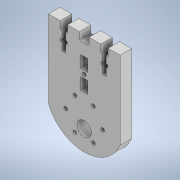
# Autodesk Inventor part: Крепление_мотора1_платформа
Saved by Autodesk Inventor 2020 (Build 240168000, 168)
## iProperties
Created: 2022-02-01
Part Number: Крепление_мотора1_платформа
Material: Типовые
Document SubType Name: Modeling
Designer: Администратор
Density: 1 g/cm^3
Appearance: По умолчанию
Autodesk Inventor part; units mm, degrees
ref_plane "YZ Plane" through (0, 0, 0) normal (1, 0, 0) x (0, 1, 0)
ref_plane "XZ Plane" through (0, 0, 0) normal (0, 1, 0) x (-1, 0, 0)
ref_plane "XY Plane" through (0, 0, 0) normal (0, 0, 1) x (1, 0, 0)
sketch "0" plane through (0, 0, 0) normal (0, 0, 1) x (1, 0, 0)
  line L0 (4.1594, 49.6005) -> (4.1594, 55.8505)
  line L1 (4.1594, 55.8505) -> (14.5761, 55.8505)
  line L2 (14.5761, 55.8505) -> (14.5761, 49.6005)
  line L3 (20.8261, 49.6005) -> (19.2636, 49.6005)
  line L4 (19.2636, 49.6005) -> (19.2636, 43.09)
  line L5 (19.2636, 33.9755) -> (16.1386, 33.9755)
  line L6 (16.1386, 33.9755) -> (16.1386, 40.4859)
  line L7 (14.8365, 43.09) -> (16.1386, 43.09)
  line L8 (20.5657, 43.09) -> (20.5657, 40.4859)
  line L9 (20.5657, 40.4859) -> (19.2636, 40.4859)
  line L10 (14.8365, 40.4859) -> (14.8365, 43.09)
  line L11 (16.1386, 43.09) -> (16.1386, 49.6005)
  line L12 (16.1386, 40.4859) -> (14.8365, 40.4859)
  line L13 (19.2636, 43.09) -> (20.5657, 43.09)
  line L14 (16.1386, 49.6005) -> (14.5761, 49.6005)
  line L15 (20.8261, 55.8505) -> (31.2428, 55.8505)
  line L16 (20.8261, 49.6005) -> (20.8261, 55.8505)
  line L17 (31.2428, 55.8505) -> (31.2428, 49.6005)
  line L18 (19.2636, 40.4859) -> (19.2636, 33.9755)
  line L19 (-31.2572, 49.6005) -> (-31.2572, 55.8505)
  line L20 (-31.2572, 55.8505) -> (-20.8406, 55.8505)
  line L21 (-14.5906, 55.8505) -> (-4.1739, 55.8505)
  line L22 (-4.1739, 55.8505) -> (-4.1739, 49.6005)
  line L23 (-3.1322, 49.6005) -> (-4.1739, 49.6005)
  line L24 (3.1178, 49.6005) -> (4.1594, 49.6005)
  line L25 (-20.8406, 55.8505) -> (-20.8406, 49.6005)
  line L26 (-14.5906, 49.6005) -> (-16.1531, 49.6005)
  line L27 (-16.1531, 49.6005) -> (-16.1531, 43.09)
  line L28 (-16.1531, 33.9755) -> (-19.2781, 33.9755)
  line L29 (-19.2781, 33.9755) -> (-19.2781, 40.4859)
  line L30 (-20.5802, 43.09) -> (-19.2781, 43.09)
  line L31 (-14.851, 43.09) -> (-14.851, 40.4859)
  line L32 (-14.851, 40.4859) -> (-16.1531, 40.4859)
  line L33 (-20.5802, 40.4859) -> (-20.5802, 43.09)
  line L34 (-19.2781, 43.09) -> (-19.2781, 49.6005)
  line L35 (-19.2781, 40.4859) -> (-20.5802, 40.4859)
  line L36 (-16.1531, 43.09) -> (-14.851, 43.09)
  line L37 (-19.2781, 49.6005) -> (-20.8406, 49.6005)
  line L38 (-14.5906, 49.6005) -> (-14.5906, 55.8505)
  line L39 (-16.1531, 40.4859) -> (-16.1531, 33.9755)
  arc A0 (-31.2572, -12.3787) -> (31.2428, -12.3787) centre (-0.0072, 0.6421) ccw
  circle A1 centre (8.0657, 5.7707) radius 1.5625
  circle A2 centre (-8.0802, 5.7707) radius 1.5625
  circle A3 centre (-16.1531, -8.212) radius 1.5625
  circle A4 centre (-8.0802, -22.1948) radius 1.5625
  circle A5 centre (8.0657, -22.1948) radius 1.5625
  circle A6 centre (16.1386, -8.212) radius 1.5625
  circle A7 centre (-0.0072, -15.5037) radius 6.25
  line L40 (31.2428, 49.6005) -> (31.2428, -12.3787)
  line L41 (-31.2572, -12.3787) -> (-31.2572, 49.6005)
  line L42 (-3.1322, 12.1005) -> (-3.1322, 22.5171)
  line L43 (-3.1322, 22.5171) -> (3.1178, 22.5171)
  line L44 (3.1178, 22.5171) -> (3.1178, 12.1005)
  line L45 (3.1178, 12.1005) -> (-3.1322, 12.1005)
  line L46 (-3.1322, 28.7671) -> (-3.1322, 39.1838)
  line L47 (3.1178, 39.1838) -> (3.1178, 28.7671)
  line L48 (3.1178, 28.7671) -> (-3.1322, 28.7671)
  circle A8 centre (-0.0072, 25.6421) radius 1.6667
  line L49 (-3.1322, 39.1838) -> (3.1178, 39.1838)
  line L50 (-3.1322, 49.6005) -> (3.1178, 49.6005)
  dimension "d0" = 12.5
  constraints: 102 end point, 9 centre point, 2 point on circle
  measures "d0" diameter of A7
sketch "Эскиз3" plane through (0, 0, 0) normal (0, 0, 1) x (1, 0, 0)
  circle A0 centre (-0.0072, -15.5037) radius 6.25
  circle A1 centre (-16.1531, -8.212) radius 1.5625
  circle A2 centre (-8.0802, 5.7707) radius 1.5625
  circle A3 centre (8.0657, 5.7707) radius 1.5625
  circle A4 centre (16.1386, -8.212) radius 1.5625
  circle A5 centre (8.0657, -22.1948) radius 1.5625
  circle A6 centre (-8.0802, -22.1948) radius 1.5625
  arc A7 (-31.2572, -12.3787) -> (31.2428, -12.3787) centre (-0.0072, 0.6421) ccw
  line L0 (-31.2572, -12.3787) -> (-31.2572, 49.6005)
  line L1 (-31.2572, 49.6005) -> (-31.2572, 55.8505)
  line L2 (-31.2572, 55.8505) -> (-20.8406, 55.8505)
  line L3 (-20.8406, 55.8505) -> (-20.8406, 49.6005)
  line L4 (-19.2781, 49.6005) -> (-20.8406, 49.6005)
  line L5 (-19.2781, 43.09) -> (-19.2781, 49.6005)
  line L6 (-20.5802, 43.09) -> (-19.2781, 43.09)
  line L7 (-20.5802, 40.4859) -> (-20.5802, 43.09)
  line L8 (-19.2781, 40.4859) -> (-20.5802, 40.4859)
  line L9 (-19.2781, 33.9755) -> (-19.2781, 40.4859)
  line L10 (-16.1531, 33.9755) -> (-19.2781, 33.9755)
  line L11 (-16.1531, 40.4859) -> (-16.1531, 33.9755)
  line L12 (-14.851, 40.4859) -> (-16.1531, 40.4859)
  line L13 (-14.851, 43.09) -> (-14.851, 40.4859)
  line L14 (-16.1531, 43.09) -> (-14.851, 43.09)
  line L15 (-16.1531, 49.6005) -> (-16.1531, 43.09)
  line L16 (-14.5906, 49.6005) -> (-16.1531, 49.6005)
  line L17 (-14.5906, 49.6005) -> (-14.5906, 55.8505)
  line L18 (-14.5906, 55.8505) -> (-4.1739, 55.8505)
  line L19 (-4.1739, 55.8505) -> (-4.1739, 49.6005)
  line L20 (-3.1322, 49.6005) -> (3.1178, 49.6005)
  line L21 (3.1178, 49.6005) -> (4.1594, 49.6005)
  line L22 (-3.1322, 49.6005) -> (-4.1739, 49.6005)
  line L23 (4.1594, 49.6005) -> (4.1594, 55.8505)
  line L24 (4.1594, 55.8505) -> (14.5761, 55.8505)
  line L25 (14.5761, 55.8505) -> (14.5761, 49.6005)
  line L26 (16.1386, 49.6005) -> (14.5761, 49.6005)
  line L27 (16.1386, 43.09) -> (16.1386, 49.6005)
  line L28 (14.8365, 43.09) -> (16.1386, 43.09)
  line L29 (14.8365, 40.4859) -> (14.8365, 43.09)
  line L30 (16.1386, 40.4859) -> (14.8365, 40.4859)
  line L31 (16.1386, 33.9755) -> (16.1386, 40.4859)
  line L32 (19.2636, 33.9755) -> (16.1386, 33.9755)
  line L33 (19.2636, 40.4859) -> (19.2636, 33.9755)
  line L34 (20.5657, 40.4859) -> (19.2636, 40.4859)
  line L35 (20.5657, 43.09) -> (20.5657, 40.4859)
  line L36 (19.2636, 43.09) -> (20.5657, 43.09)
  line L37 (19.2636, 49.6005) -> (19.2636, 43.09)
  line L38 (20.8261, 49.6005) -> (19.2636, 49.6005)
  line L39 (20.8261, 49.6005) -> (20.8261, 55.8505)
  line L40 (20.8261, 55.8505) -> (31.2428, 55.8505)
  line L41 (31.2428, 49.6005) -> (31.2428, -12.3787)
  line L42 (3.1178, 22.5171) -> (3.1178, 12.1005)
  circle A8 centre (-0.0072, 25.6421) radius 1.6667
  line L43 (3.1178, 28.7671) -> (-3.1322, 28.7671)
  line L44 (-3.1322, 28.7671) -> (-3.1322, 39.1838)
  line L45 (-3.1322, 39.1838) -> (3.1178, 39.1838)
  line L46 (3.1178, 39.1838) -> (3.1178, 28.7671)
  line L47 (-3.1322, 22.5171) -> (3.1178, 22.5171)
  line L48 (-3.1322, 12.1005) -> (-3.1322, 22.5171)
  line L49 (3.1178, 12.1005) -> (-3.1322, 12.1005)
  line L50 (31.2428, 55.8505) -> (31.2428, 49.6005)
  line L51 (31.2428, 55.8505) -> (31.2428, -12.3787)
  line L52 (20.8261, 55.8505) -> (31.2428, 55.8505)
  line L53 (20.8261, 55.8505) -> (20.8261, 49.6005)
  line L54 (19.2636, 49.6005) -> (20.8261, 49.6005)
  line L55 (19.2636, 43.09) -> (19.2636, 49.6005)
  line L56 (20.5657, 43.09) -> (19.2636, 43.09)
  line L57 (20.5657, 43.09) -> (20.5657, 40.4859)
  line L58 (20.5657, 40.4859) -> (19.2636, 40.4859)
  line L59 (19.2636, 40.4859) -> (19.2636, 33.9755)
  line L60 (16.1386, 33.9755) -> (19.2636, 33.9755)
  line L61 (16.1386, 40.4859) -> (16.1386, 33.8824)
  line L62 (14.8365, 40.4859) -> (16.1386, 40.4859)
  line L63 (14.8365, 43.09) -> (14.8365, 40.4859)
  line L64 (16.1386, 43.09) -> (14.8365, 43.09)
  line L65 (16.1386, 49.6005) -> (16.1386, 43.09)
  line L66 (16.1386, 49.6005) -> (14.5761, 49.6005)
  line L67 (14.5761, 49.6005) -> (14.5761, 55.8505)
  line L68 (4.1594, 55.8505) -> (14.5761, 55.8505)
  line L69 (4.1594, 55.8505) -> (4.1594, 49.6005)
  line L70 (-3.1322, 39.1838) -> (3.1178, 39.1838)
  line L71 (3.1178, 39.1838) -> (3.1178, 28.7671)
  line L72 (3.1178, 28.7671) -> (-3.1322, 28.7671)
  line L73 (-3.1322, 28.7671) -> (-3.1322, 39.1838)
  line L74 (-3.1322, 22.5171) -> (3.1178, 22.5171)
  line L75 (3.1178, 22.5171) -> (3.1178, 12.1005)
  line L76 (3.1178, 12.1005) -> (-3.1322, 12.1005)
  line L77 (-3.1322, 12.1005) -> (-3.1322, 22.5171)
  circle A9 centre (-0.0072, -15.5037) radius 6.25
  circle A10 centre (16.1386, -8.212) radius 1.5625
  circle A11 centre (8.0657, 5.7707) radius 1.5625
  circle A12 centre (8.0657, -22.1948) radius 1.5625
  circle A13 centre (-8.0802, 5.7707) radius 1.5625
  circle A14 centre (-16.1531, -8.212) radius 1.5625
  circle A15 centre (-8.0802, -22.1948) radius 1.5625
  line L78 (-14.5906, 55.8505) -> (-14.5906, 49.6005)
  line L79 (-20.8406, 49.6005) -> (-20.8406, 55.8505)
  line L80 (-14.851, 43.09) -> (-14.851, 40.4859)
  line L81 (-20.5802, 40.4859) -> (-20.5802, 43.09)
  line L82 (-16.1531, 33.9755) -> (-19.2781, 33.9755)
  line L83 (-20.8406, 55.8505) -> (-20.5802, 55.8505)
  line L84 (-14.851, 55.8505) -> (-14.5906, 55.8505)
  line L85 (-14.5906, 49.6005) -> (-16.1531, 49.6005)
  line L86 (-19.2781, 49.6005) -> (-20.8406, 49.6005)
  line L87 (-19.2781, 33.9755) -> (-19.2781, 40.4859)
  line L88 (-19.2781, 43.09) -> (-19.2781, 49.6005)
  line L89 (-16.1531, 49.6005) -> (-16.1531, 43.09)
  line L90 (-16.1531, 40.4859) -> (-16.1531, 33.9755)
  line L91 (-20.5802, 43.09) -> (-19.2781, 43.09)
  line L92 (-16.1531, 43.09) -> (-14.851, 43.09)
  line L93 (-14.851, 40.4859) -> (-16.1531, 40.4859)
  line L94 (-19.2781, 40.4859) -> (-20.5802, 40.4859)
  line L95 (-31.2572, 55.8505) -> (-31.2572, -12.3787)
  line L96 (-31.2572, 55.8505) -> (-20.5802, 55.8505)
  line L97 (-14.851, 55.8505) -> (-4.1739, 55.8505)
  line L98 (-4.1739, 55.8505) -> (-4.1739, 49.6005)
  line L99 (-4.1739, 49.6005) -> (4.1594, 49.6005)
  circle A16 centre (-0.0072, 25.6421) radius 1.6667
  arc A17 (-31.2572, -12.3787) -> (31.2428, -12.3787) centre (-0.0072, 0.6421) ccw
  point P0 (0, 0)
  point P1 (-0.0072, 12.1005)
  point P2 (3.1178, 17.3088)
  dimension "d1" = 33.8542
  dimension "d2" = 12.5
  constraints: 204 end point, 49 horizontal, 39 vertical, 19 parallel, 18 centre point, 15 collinear, 14 perpendicular, 8 coincident, 8 concentric, 4 point on circle, 3 point on line, 2 midpoint, 98 other
  measures "d1" radius of A7
  measures "d2" diameter of A0
extrude "Выдавливание1" add sketch "Эскиз3" along normal blind 10
